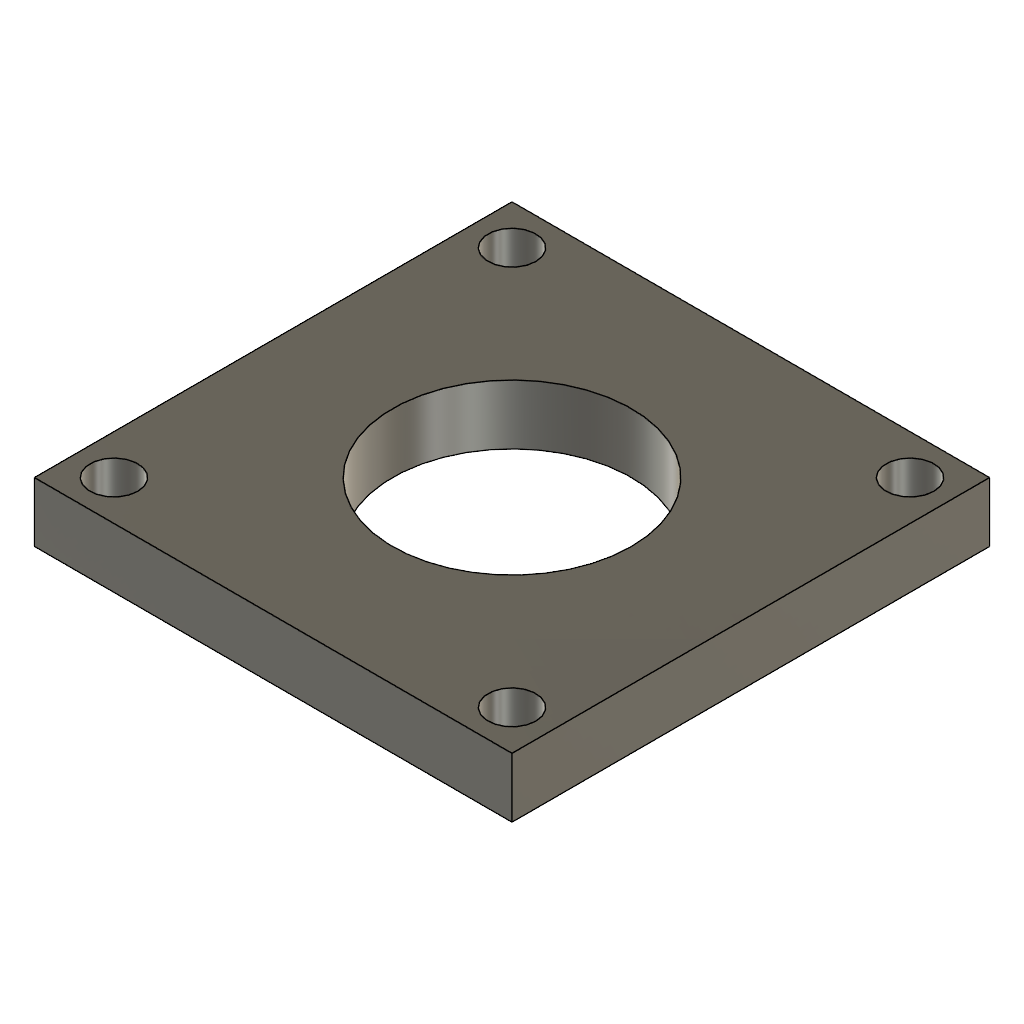
VTX_Mount (Autodesk Fusion 360 design; units mm, degrees)
part number: 2026-09-21-21-38-08-263
Autodesk Fusion 360 part; units mm, degrees
sketch "Sketch1" plane through (0, 0, 0) normal (0, 0, 1) x (1, 0, 0)
  line L0 (12, -12) -> (-12, -12)
  line L1 (-12, -12) -> (-12, 12)
  line L2 (-12, 12) -> (12, 12)
  line L3 (12, 12) -> (12, -12)
  line L4 (12, -12) -> (-12, 12) construction
  line L5 (-12, -12) -> (12, 12) construction
  dimension "d1" = 24
  dimension "d2" = 24
  constraint horizontal L0
  constraint perpendicular L0 L1
  constraint parallel L0 L2
  constraint parallel L1 L3
  constraint coincident L4 origin
  constraint coincident L5 origin
  measures "d1" distance of L0.end L1.end
  measures "d2" distance of L1.end L2.end
extrude "Extrude1" add sketch "Sketch1" along normal blind 3
sketch "Sketch2" plane through (0, 0, 3) normal (0, 0, 1) x (-1, 0, 0)
  line L0 (-12, -12) -> (12, -12)
  line L1 (12, -12) -> (12, 12)
  line L2 (12, 12) -> (-12, 12)
  line L3 (-12, 12) -> (-12, -12)
  circle A0 centre (10, -10) radius 1.1
  circle A1 centre (-10, -10) radius 1.1
  circle A2 centre (10, 10) radius 1.1
  circle A3 centre (-10, 10) radius 1.1
  dimension "d5" = 2.2
  dimension "d6" = 2.2
  dimension "d7" = 2.2
  dimension "d8" = 2.2
  dimension "d9" = 10
  dimension "d10" = 10
  dimension "d11" = 10
  dimension "d12" = 10
  dimension "d13" = 10
  dimension "d14" = 10
  dimension "d15" = 10
  dimension "d16" = 10
  measures "d5" diameter of A0
  measures "d6" diameter of A1
  measures "d7" diameter of A2
  measures "d8" diameter of A3
  measures "d9" vertical distance of origin A0.centre
  measures "d10" vertical distance of origin A3.centre
  measures "d11" horizontal distance of origin A3.centre
  measures "d12" horizontal distance of origin A1.centre
  measures "d13" vertical distance of origin A1.centre
  measures "d14" vertical distance of origin A2.centre
  measures "d15" horizontal distance of origin A2.centre
  measures "d16" vertical distance of origin A0.centre
extrude "Extrude2" cut sketch "Sketch2" against normal through all contours A0 | A1 | A2 | A3
sketch "Sketch3" plane through (0, 0, 3) normal (0, 0, 1) x (-1, 0, 0)
  circle A0 centre (10, -10) radius 1.1
  circle A1 centre (10, 10) radius 1.1
  circle A2 centre (-10, -10) radius 1.1
  circle A3 centre (-10, 10) radius 1.1
  line L0 (-12, -12) -> (12, -12)
  line L1 (12, -12) -> (12, 12)
  line L2 (12, 12) -> (-12, 12)
  line L3 (-12, 12) -> (-12, -12)
  circle A4 centre (0, 0) radius 6
  dimension "d18" = 12
  constraint coincident A4.centre origin
  measures "d18" diameter of A4
extrude "Extrude3" cut sketch "Sketch3" against normal blind 6 contours A4
sketch "Sketch4" plane through (0, 0, 3) normal (0, 0, 1) x (-1, 0, 0)
  circle A0 centre (0, 0) radius 6
  circle A1 centre (10, -10) radius 1.1
  circle A2 centre (10, 10) radius 1.1
  circle A3 centre (-10, -10) radius 1.1
  circle A4 centre (-10, 10) radius 1.1
  line L0 (-12, -12) -> (12, -12)
  line L1 (12, -12) -> (12, 12)
  line L2 (12, 12) -> (-12, 12)
  line L3 (-12, 12) -> (-12, -12)
  circle A5 centre (10, -10) radius 1.2
  circle A6 centre (-10, -10) radius 1.2
  circle A7 centre (10, 10) radius 1.2
  circle A8 centre (-10, 10) radius 1.2
  dimension "d21" = 2.4
  dimension "d22" = 2.4
  dimension "d23" = 2.4
  dimension "d24" = 2.4
  constraint concentric A1 A5
  constraint concentric A3 A6
  constraint concentric A2 A7
  constraint concentric A4 A8
  measures "d21" diameter of A5
  measures "d22" diameter of A6
  measures "d23" diameter of A7
  measures "d24" diameter of A8
extrude "Extrude4" cut sketch "Sketch4" against normal blind 5 contours A5 | A6 | A7 | A8
named bodies: "VTX_Mount_body"
